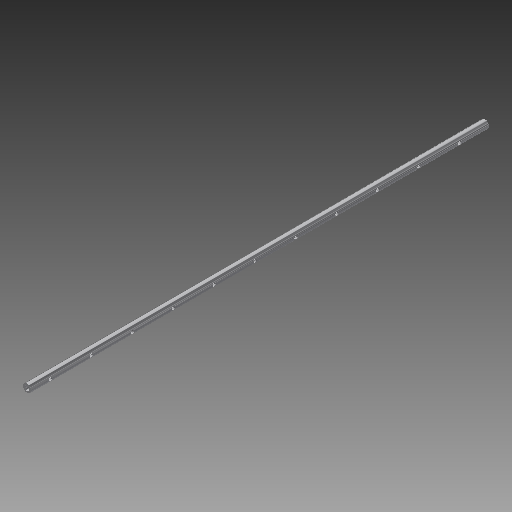
# Autodesk Inventor part: 202-17
Saved by Autodesk Inventor 2019 (Build 230136000, 136)
## iProperties
Company: Autodesk Inc.
Created: 2007-11-04
Part Number: 202-17
Document SubType Name: Modeling
Designer: Autodesk Inc.
Density: 2.7 g/cm^3
Mass: 9.29539 g
Surface Area: 70.6339 cm^2
Volume: 3.44274 cm^3
Material: Aluminum-6061
Description: WIRE CONNECTOR BAR
Appearance: Aluminum - Polished
Component Category: Back Component
Author: Inventor
Autodesk Inventor part; units mm, degrees
ref_plane "YZ Plane" through (0, 0, 0) normal (1, 0, 0) x (0, 1, 0)
ref_plane "XZ Plane" through (0, 0, 0) normal (0, 1, 0) x (-1, 0, 0)
ref_plane "XY Plane" through (0, 0, 0) normal (0, 0, 1) x (1, 0, 0)
sketch "Sketch1" plane through (0, 0, 0) normal (0, 0, 1) x (1, 0, 0)
  circle A0 centre (0, 0) radius 2.5
  circle A1 centre (0, 0) radius 1.5
  dimension "d0" = 5
  dimension "d1" = 3
  constraints: 2 centre point, 2 coincident
  measures "d0" diameter of A0
  measures "d1" diameter of A1
extrude "Extrusion1" add sketch "Sketch1" along normal mid plane 280
sketch "Sketch2" plane through (0, 0, 0) normal (1, 0, 0) x (0, 1, 0)
  line L0 (-1.5, 140) -> (1.5, 140) projected
  line L1 (-2.5, 140) -> (2.5, 140) projected
  line L2 (0, 140) -> (0, 128)
  circle A0 centre (0, 128) radius 1.025
  circle A1 centre (0, 103) radius 1.025
  circle A2 centre (0, 78) radius 1.025
  circle A3 centre (0, 53) radius 1.025
  circle A4 centre (0, 28) radius 1.025
  circle A5 centre (0, 3) radius 1.025
  circle A6 centre (0, -22) radius 1.025
  circle A7 centre (0, -47) radius 1.025
  circle A8 centre (0, -72) radius 1.025
  circle A9 centre (0, -97) radius 1.025
  circle A10 centre (0, -122) radius 1.025
  point P0 (0, 0)
  dimension "d4" = 12
  dimension "d5" = 2.05
  dimension "d8" = 25
  constraints: 11 centre point, 2 end point, 1 coincident, 1 midpoint, 1 perpendicular, 1 vertical, 20 other
  measures "d4" distance of L2.start L2.end
  measures "d5" diameter of A0
  measures "d8" distance of A0.centre A1.centre
extrude "Extrusion2" cut sketch "Sketch2" along normal through all both and the other way through all
body "Solid1"
